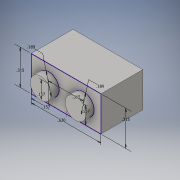
# Autodesk Inventor part: bricks
Saved by Autodesk Inventor 2016 (Build 200138000, 138)
## iProperties
Created: 2018-02-13
Part Number: bricks
Material: Generic
Document SubType Name: Modeling
Designer: sun01147
Density: 1 g/cm^3
Appearance: Default
Author: sun01147
Autodesk Inventor part; units mm, degrees
ref_plane "YZ Plane" through (0, 0, 0) normal (1, 0, 0) x (0, 1, 0)
ref_plane "XZ Plane" through (0, 0, 0) normal (0, 1, 0) x (-1, 0, 0)
ref_plane "XY Plane" through (0, 0, 0) normal (0, 0, 1) x (1, 0, 0)
sketch "Top" plane through (0, 0, 0) normal (0, 0, 1) x (1, 0, 0)
  line L0 (0, 8) -> (0, 0)
  line L1 (0, 0) -> (16, 0)
  line L2 (16, 0) -> (16, 8)
  line L3 (0, 8) -> (16, 8)
  circle A0 centre (4, 4) radius 2.4
  circle A1 centre (12, 4) radius 2.4
  point P0 (8, 0)
  dimension "d0" = 16
  dimension "d1" = 8
  dimension "d2" = 8
  dimension "d3" = 4.8
  dimension "d4" = 4.8
  dimension "d5" = 8
  dimension "d6" = 4
  dimension "d7" = 4
  dimension "d8" = 4
  constraints: 8 end point, 2 centre point, 2 perpendicular, 1 midpoint, 1 vertical
  measures "d0" distance of L0.end L1.end
  measures "d1" distance of L0.start L0.end
  measures "d2" distance of L1.end L2.end
  measures "d3" diameter of A0
  measures "d4" diameter of A1
  measures "d5" distance of A1.centre A0.centre
  measures "d6" distance from line of L1 A0.centre
  measures "d7" distance from line of L1 A1.centre
  measures "d8" distance from line of L0 A0.centre
extrude "Extrusion1" add sketch "Top" against normal blind 9.6
extrude "Extrusion2" add sketch "Top" along normal blind 1.8 contours A0 | A1
sketch "Sketch2" plane through (0, 0, -9.6) normal (0, 0, -1) x (-1, 0, 0)
  line L0 (0, 8) -> (-16, 8) projected
  line L1 (-16, 0) -> (0, 0) projected
  line L2 (-16, 8) -> (0, 8)
  line L3 (0, 8) -> (0, 0)
  line L4 (0, 0) -> (-16, 0)
  line L5 (-16, 0) -> (-16, 8)
  circle A0 centre (-12, 4) radius 2.3827
  circle A1 centre (-4, 4) radius 2.4067
  dimension "d13" = 4
  dimension "d14" = 4
  dimension "d15" = 8
  dimension "d16" = 4
  dimension "d17" = 4.7654
  dimension "d18" = 4.8133
  constraints: 8 end point, 2 centre point, 2 parallel, 1 horizontal, 1 perpendicular
  measures "d13" distance from line of L1 A0.centre
  measures "d14" distance from line of L5 A0.centre
  measures "d15" distance of A1.centre A0.centre
  measures "d16" distance from line of L3 A1.centre
  measures "d17" diameter of A0
  measures "d18" diameter of A1
extrude "Extrusion3" add sketch "Sketch2" against normal blind 1.8 contours A0 | A1
sketch "Sketch3" plane through (0, 0, -9.6) normal (0, 0, -1) x (-1, 0, 0)
  line L0 (-16, 8) -> (-16, 0) projected
  line L1 (0, 0) -> (0, 8) projected
  line L2 (-16, 8) -> (0, 8)
  line L3 (0, 8) -> (0, 0)
  line L4 (-16, 0) -> (0, 0) projected
  line L5 (0, 0) -> (-16, 0)
  line L6 (-16, 0) -> (-16, 8)
  line L7 (-14.9, 6.9) -> (-1.1, 6.9)
  line L8 (-1.1, 6.9) -> (-1.1, 1.1)
  line L9 (-1.1, 1.1) -> (-14.9, 1.1)
  line L10 (-14.9, 1.1) -> (-14.9, 6.9)
  dimension "d21" = 1.1
  dimension "d22" = 1.1
  dimension "d23" = 1.1
  dimension "d24" = 1.1
  constraints: 16 end point, 4 equal length, 3 perpendicular, 1 horizontal
  measures "d21" distance from line of L2 L7.start
  measures "d22" distance between parallel lines of L0 L10
  measures "d23" distance between parallel lines of L4 L9
  measures "d24" distance between parallel lines of L1 L8
extrude "Extrusion4" cut sketch "Sketch3" against normal blind 1.8 contours L7 L8 L9 L10
body "Solid1"
